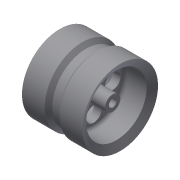
# Autodesk Inventor part: Tank Wheel
Saved by Autodesk Inventor 2015 (Build 190159000, 159)
## iProperties
Created: 2015-03-12
Part Number: Tank Wheel
Material: Generic
Document SubType Name: Modeling
Designer: james_000
Density: 1 g/cm^3
Appearance: Default
Author: james_000
Autodesk Inventor part; units mm, degrees
ref_plane "YZ Plane" through (0, 0, 0) normal (1, 0, 0) x (0, 1, 0)
ref_plane "XZ Plane" through (0, 0, 0) normal (0, 1, 0) x (-1, 0, 0)
ref_plane "XY Plane" through (0, 0, 0) normal (0, 0, 1) x (1, 0, 0)
sketch "Sketch1" plane through (0, 0, 0) normal (0, 0, 1) x (1, 0, 0)
  line L0 (6, 0) -> (6, 2)
  line L1 (6, 0) -> (1, 0)
  line L2 (6, 2) -> (-6, 2)
  line L3 (-6, 2) -> (-6, 0)
  line L4 (-6, 0) -> (-1, 0)
  line L5 (-8, -8) -> (-7, -6)
  line L6 (8, -8) -> (7, -6)
  line L7 (-7, -6) -> (-2, -6)
  line L8 (-1, 0) -> (-1, -5)
  arc A0 (-2, -6) -> (-1, -5) centre (-2, -5) ccw
  line L9 (-8, -8) -> (-2, -8)
  line L10 (-2, -8) -> (-1, -7)
  line L11 (-1, -7) -> (1, -7)
  line L12 (1, -7) -> (2, -8)
  line L13 (2, -8) -> (8, -8)
  line L14 (1, 0) -> (1, -5)
  line L15 (7, -6) -> (2, -6)
  arc A1 (1, -5) -> (2, -6) centre (2, -5) ccw
  point P0 (0, 0)
  dimension "d0" = 6
  dimension "d1" = 2
  dimension "d3" = 5
  dimension "d6" = 12
  dimension "d7" = 2
  dimension "d8" = 5
  dimension "d26" = 5
  dimension "d27" = 5
  dimension "d28" = 6
  dimension "d29" = 5
  dimension "d30" = 5
  constraints: 32 end point, 5 horizontal, 4 point on circle, 3 perpendicular, 2 centre point, 2 vertical, 1 collinear, 1 parallel, 1 point on line
  measures "d0" distance of point (0, 0) L0.start
  measures "d1" distance of L0.start L0.end
  measures "d3" distance of L0.start L1.end
  measures "d6" distance of L0.end L2.end
  measures "d7" distance of L2.end L3.end
  measures "d8" distance of L3.end L4.end
  measures "d26" distance of L5.end L7.end
  measures "d27" distance of L4.end L8.end
  measures "d28" distance of L5.start L9.end
  measures "d29" distance of L1.end L14.end
  measures "d30" distance of L6.end L15.end
revolve "Revolution1" add sketch "Sketch1" angle 360 about axis through (6, 2, 0) along (-1, 0, 0)
sketch "Sketch2" plane through (1, 2, 0) normal (1, 0, 0) x (0, 0, -1)
  circle A0 centre (0, 0) radius 8 projected
  line L0 (0, 8) -> (0, 5)
  line L1 (-8, 0) -> (-5, 0)
  line L2 (0, -8) -> (0, -5)
  line L3 (8, 0) -> (5, 0)
  point P0 (0, -2)
  dimension "d15" = 3
  dimension "d16" = 3
  dimension "d17" = 3
  dimension "d18" = 3
  constraints: 8 end point, 4 point on circle, 2 horizontal, 2 vertical
  measures "d15" distance of L0.start L0.end
  measures "d16" distance of L1.start L1.end
  measures "d17" distance of L2.start L2.end
  measures "d18" distance of L3.start L3.end
hole "Hole1" [suppressed]
sketch "Sketch3" plane through (1, 2, 0) normal (1, 0, 0) x (0, 0, -1)
  line L0 (0, 2.0456) -> (0, 5.0456)
  circle A0 centre (0, 0) radius 2 projected
  line L1 (-2, 0) -> (-5, 0)
  line L2 (0, -2) -> (0, -5)
  line L3 (2, 0) -> (5, 0)
  dimension "d31" = 3
  dimension "d32" = 3
  dimension "d33" = 3
  dimension "d34" = 3
  constraints: 8 end point, 2 horizontal, 2 point on circle, 2 vertical
  measures "d31" distance of L0.start L0.end
  measures "d32" distance of L1.start L1.end
  measures "d33" distance of L2.start L2.end
  measures "d34" distance of L3.start L3.end
hole "Hole2" at (1, 7.0456, 0) at (1, 2, -5) at (1, -3, 0) at (1, 2, 5) direction (-1, 0, 0) diameter 4 depth 8
sketch "Sketch5" plane through (6, 2, 0) normal (1, 0, 0) x (0, 0, -1)
  point P0 (0, 0)
  point P1 (0, 0)
  constraints: 1 coincident
hole "Hole3" at (6, 2, 0) direction (-1, 0, 0) diameter 2 depth 20
body "Solid1"
